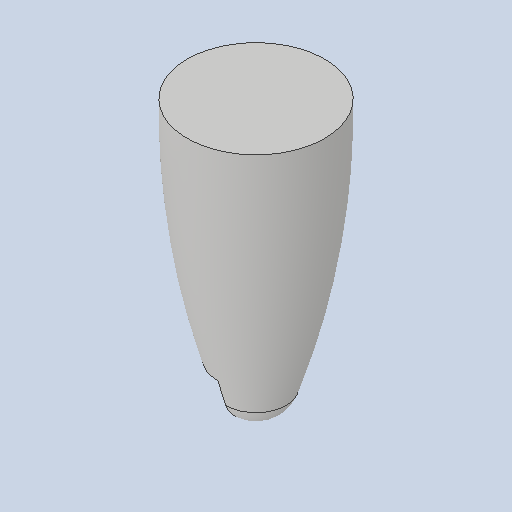
# Autodesk Inventor part: ч ASY human dummy 01
Saved by Autodesk Inventor 2024.2 (Build 282272000, 272)
## iProperties
Created: 2019-08-19
Part Number: ч ASY human dummy 01
Material: Типовые
Document SubType Name: Modeling
Designer: admin
Density: 1 g/cm^3
Appearance: По умолчанию
Author: admin
Autodesk Inventor part; units mm, degrees
ref_plane "YZ Plane" through (0, 0, 0) normal (1, 0, 0) x (0, 1, 0)
ref_plane "XZ Plane" through (0, 0, 0) normal (0, 1, 0) x (-1, 0, 0)
ref_plane "XY Plane" through (0, 0, 0) normal (0, 0, 1) x (1, 0, 0)
sketch "Эскиз1" plane through (0, 0, 0) normal (0, 0, 1) x (1, 0, 0)
  arc A0 (-49.6078, 6.25) -> (0, -50) centre (0, 0) ccw construction
  arc A1 (0, -225) -> (-23.7255, -257.8804) centre (0, -250) ccw construction
  arc A2 (-49.6078, 6.25) -> (-54.25, -60) centre (545.6862, -68.75) ccw construction
  line L0 (0, 0) -> (0, -225)
  line L1 (0, -60) -> (-54.25, -60)
  line L2 (0, -225) -> (0, -250)
  line L3 (0, -250) -> (0, -275)
  arc A3 (0, -275) -> (0, -225) centre (0, -250) ccw construction
  arc A4 (-23.7255, -257.8804) -> (0, -275) centre (0, -250) ccw
  line L4 (0, 0) -> (0, 50) construction
  arc A5 (0, 50) -> (-49.6078, 6.25) centre (0, 0) ccw
  arc A6 (0, -50) -> (0, 50) centre (0, 0) ccw
  arc A7 (-54.25, -60) -> (-23.7255, -257.8804) centre (545.6862, -68.75) ccw
  dimension "d0" = 100
  dimension "d1" = 50
  dimension "d2" = 250
  dimension "d3" = 600
  dimension "d4" = 60
  constraints: 16 point on circle, 10 end point, 8 centre point, 4 vertical, 2 point on line, 2 tangent, 1 coincident, 1 horizontal
  measures "d0" diameter of A0
  measures "d1" diameter of A1
  measures "d2" distance of L2.end point (0, 0)
  measures "d3" radius of A2
  measures "d4" distance from line of point (0, 0) L1
revolve "Вращение1" add sketch "Эскиз1" angle 360 about axis through (0, 0, 0) along (0, -1, 0)
sketch "Эскиз2" plane through (0, 0, 0) normal (1, 0, 0) x (0, 1, 0)
  line L0 (-257.8804, -23.7255) -> (-257.8804, 23.7255) projected
  line L1 (-257.8804, -23.7255) -> (-257.8804, 23.7255) projected
  line L2 (-60, -54.25) -> (-60, 54.25) projected
  circle A0 centre (-250, 0) radius 25
  line L3 (-250, 25) -> (-250, -25)
  point P0 (0, 0)
  dimension "d6" = 50
  constraints: 4 point on circle, 2 end point, 1 centre point, 1 vertical
  measures "d6" diameter of A0
revolve "Вращение2" cut sketch "Эскиз2" angle 180 about axis through (0, -250, 25) along (0, 0, -1) contours A0 L0 | L0 A0 L3
sketch "Эскиз3" plane through (0, 0, 0) normal (0, 0, 1) x (1, 0, 0)
  line L0 (0, -275) -> (0, -257.8804) projected
  arc A0 (-54.25, -60) -> (-23.7255, -257.8804) centre (545.6862, -68.75) ccw projected
  line L1 (0, -275) -> (-30, -275)
  line L2 (-30, -275) -> (-30, -237.8221)
  line L3 (-30, -237.8221) -> (0, -237.8221)
  line L4 (0, -237.8221) -> (0, -275)
  point P0 (0, 0)
  dimension "d8" = 30
  constraints: 8 end point, 2 parallel, 1 horizontal, 1 perpendicular, 1 point on circle
  measures "d8" distance of L2.end L3.end
extrude "Выдавливание1" cut sketch "Эскиз3" along normal through all both and the other way through all
